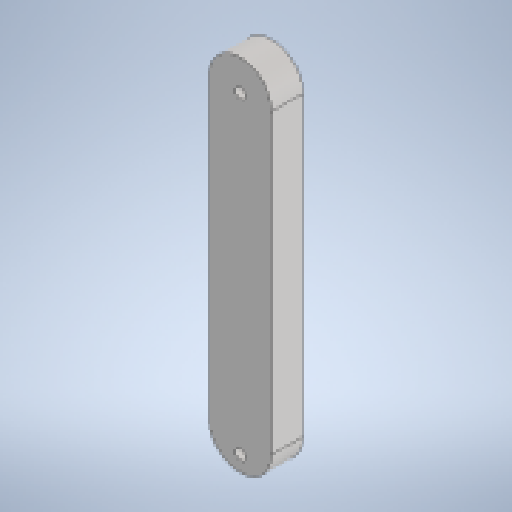
# Autodesk Inventor part: шатун
Saved by Autodesk Inventor 2023.1 (Build 271208000, 208)
## iProperties
Created: 2024-12-17
Part Number: шатун
Material: Типовые
Document SubType Name: Modeling
Designer: DELL
Density: 1 g/cm^3
Appearance: По умолчанию
Author: DELL
Autodesk Inventor part; units mm, degrees
ref_plane "YZ Plane" through (0, 0, 0) normal (1, 0, 0) x (0, 1, 0)
ref_plane "XZ Plane" through (0, 0, 0) normal (0, 1, 0) x (-1, 0, 0)
ref_plane "XY Plane" through (0, 0, 0) normal (0, 0, 1) x (1, 0, 0)
sketch "Эскиз1" plane through (0, 0, 0) normal (0, 0, 1) x (1, 0, 0)
  circle A0 centre (0, 0) radius 5 construction
  circle A1 centre (0, 0) radius 1.575 projected
  line L0 (343.1024, 82) -> (-136.8976, 82) construction
  line L1 (0, -5) -> (0, 110) construction
  line L2 (10, 5) -> (10, 100)
  line L3 (-10, 100) -> (-10, 5)
  arc A2 (-10, 5) -> (10, 5) centre (0, 5) ccw
  arc A3 (10, 100) -> (-10, 100) centre (0, 100) ccw
  circle A4 centre (0, 100) radius 1.575
  point P0 (0, 0)
  point P1 (0, 52.5)
  dimension "d0" = 115
  dimension "d1" = 20
  constraints: 8 end point, 6 point on circle, 4 tangent, 3 centre point, 2 point on line, 1 coincident, 1 midpoint, 1 parallel, 1 vertical, 1 vertical alignment, 1 other
  measures "d0" distance of L1.start L1.end
  measures "d1" diameter of A3
extrude "Выдавливание1" add sketch "Эскиз1" along normal blind 10
